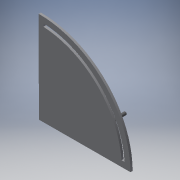
# Autodesk Inventor part: arco base
Saved by Autodesk Inventor 2019 (Build 230136000, 136)
## iProperties
Created: 2018-07-24
Part Number: arco base
Material: Genérico
Document SubType Name: Modeling
Designer: Ernandes
Density: 1 g/cm^3
Appearance: Padrão
Author: Ernandes
Autodesk Inventor part; units mm, degrees
ref_plane "YZ Plane" through (0, 0, 0) normal (1, 0, 0) x (0, 1, 0)
ref_plane "XZ Plane" through (0, 0, 0) normal (0, 1, 0) x (-1, 0, 0)
ref_plane "XY Plane" through (0, 0, 0) normal (0, 0, 1) x (1, 0, 0)
sketch "Esboço1" plane through (0, 0, 0) normal (0, 0, 1) x (1, 0, 0)
  arc A0 (189.4753, 14.1106) -> (10.246, 189.7235) centre (0, 0) ccw
  line L0 (0, 0) -> (-0.575, 189.9991) construction
  line L1 (0, 0) -> (189.9991, 0.575) construction
  arc A1 (196.456, 14.6304) -> (10.6234, 196.7134) centre (0, 0) ccw
  arc A2 (209.999, 0.6355) -> (-0.6355, 209.999) centre (0, 0) ccw
  line L2 (0, 0) -> (-0.6355, 209.999)
  line L3 (0, 0) -> (209.999, 0.6355)
  line L4 (10.246, 189.7235) -> (10.6234, 196.7134)
  line L5 (189.4753, 14.1106) -> (196.456, 14.6304)
  dimension "d3" = 190
  dimension "d4" = 90
  dimension "d5" = 197
  dimension "d6" = 210
  constraints: 12 end point, 6 point on circle, 3 centre point, 2 coincident, 2 collinear
  measures "d3" radius of A0
  measures "d4" angle of L1 L0
  measures "d5" radius of A1
  measures "d6" radius of A2
extrude "Extrusão1" add sketch "Esboço1" along normal blind 5
sketch "Esboço2" plane through (0, 0, 0) normal (0, 0, -1) x (-1, 0, 0)
  line L0 (0.6355, 209.999) -> (0, 0) projected
  circle A0 centre (-172.9136, 86.6806) radius 3.4935
  constraints: 1 centre point
extrude "Extrusão2" add sketch "Esboço2" along normal blind 20 and the other way blind 5
thread "Rosca1" size "M7x1" class "6g" standard "ANSI Metric M Profile" full length
move faces "Mover1" translate (0, 0, 5) faces at (171.993, 86.7732, -20)
